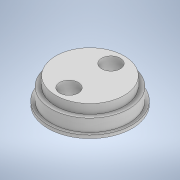
# Autodesk Inventor part: RotorShaft3
Saved by Autodesk Inventor 2021 (Build 250183000, 183)
## iProperties
Created: 2022-08-31
Part Number: RotorShaft3
Material: Ogólny
Document SubType Name: Modeling
Designer: MicnedSQ
Density: 1 g/cm^3
Appearance: Domyślna
Author: MicnedSQ
Autodesk Inventor part; units mm, degrees
ref_plane "YZ Plane" through (0, 0, 0) normal (1, 0, 0) x (0, 1, 0)
ref_plane "XZ Plane" through (0, 0, 0) normal (0, 1, 0) x (-1, 0, 0)
ref_plane "XY Plane" through (0, 0, 0) normal (0, 0, 1) x (1, 0, 0)
sketch "Szkic1" plane through (0, 0, 0) normal (0, 1, 0) x (-1, 0, 0)
  circle A0 centre (0, 0) radius 13.5
  dimension "d0" = 27
  constraints: 1 centre point, 1 coincident
  measures "d0" diameter of A0
extrude "Wyciągnięcie proste1" add sketch "Szkic1" along normal blind 1
sketch "Szkic2" plane through (0, 1, 0) normal (0, 1, 0) x (1, 0, 0)
  circle A0 centre (0, 0) radius 12.5
  dimension "d3" = 25
  constraints: 1 centre point, 1 coincident
  measures "d3" diameter of A0
extrude "Wyciągnięcie proste2" add sketch "Szkic2" along normal blind 4
sketch "Szkic3" plane through (0, 5, 0) normal (0, 1, 0) x (1, 0, 0)
  arc A0 (2.12, 1.59) -> (2.12, -1.59) centre (0, 0) ccw
  line L0 (2.12, -1.59) -> (2.12, 1.59)
  dimension "d6" = 5.3
  dimension "d7" = 2.12
  constraints: 2 end point, 2 point on circle, 1 centre point, 1 coincident, 1 vertical
  measures "d6" diameter of A0
  measures "d7" distance from line of L0 point (0, 0)
extrude "Wyciągnięcie proste3" cut sketch "Szkic3" against normal through all
sketch "Szkic4" plane through (0, 5, 0) normal (0, 1, 0) x (1, 0, 0)
  circle A0 centre (0, -6.75) radius 3
  point P0 (0, 0)
  dimension "d10" = 6
  constraints: 1 centre point
  measures "d10" diameter of A0
extrude "Wyciągnięcie proste4" cut sketch "Szkic4" against normal blind 2.5
sketch "Szkic5" plane through (0, 2.5, 6.75) normal (0, 1, 0) x (1, 0, 0)
  circle A0 centre (0, 0) radius 1.6
  point P0 (0, 6.75)
  dimension "d13" = 3.2
  constraints: 1 centre point
  measures "d13" diameter of A0
extrude "Wyciągnięcie proste5" cut sketch "Szkic5" against normal blind 3.5
pattern_circular "Szyk kołowy1" count 2 over 360 about axis through (0, 1, 0) along (0, 1, 0) of "Wyciągnięcie proste4", "Wyciągnięcie proste5"
sketch "Szkic6" plane through (0, 5, 0) normal (0, 1, 0) x (1, 0, 0)
  circle A0 centre (0, 0) radius 11
  circle A1 centre (0, 6.75) radius 3 projected
  circle A2 centre (0, 6.75) radius 3
  circle A3 centre (0, -6.75) radius 3 projected
  circle A4 centre (0, -6.75) radius 3
  arc A5 (2.12, 1.59) -> (2.12, -1.59) centre (0, 0) ccw
  line L0 (2.12, 1.59) -> (2.12, -1.59) projected
  line L1 (2.12, -1.59) -> (2.12, 1.59)
  dimension "d19" = 22
  constraints: 4 centre point, 4 coincident, 2 end point, 2 point on circle, 1 collinear
  measures "d19" diameter of A0
extrude "Wyciągnięcie proste6" add sketch "Szkic6" along normal blind 3
sketch "Szkic7" plane through (0, 8, 0) normal (0, 1, 0) x (1, 0, 0)
  arc A0 (2.12, 1.59) -> (2.12, -1.59) centre (0, 0) ccw
  line L0 (2.12, 1.59) -> (2.12, -1.59) projected
  line L1 (2.12, -1.59) -> (2.12, 1.59)
  constraints: 2 end point, 2 point on circle, 1 centre point, 1 coincident, 1 collinear
extrude "Wyciągnięcie proste7" add sketch "Szkic7" against normal blind 0.5
